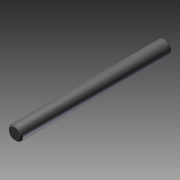
# Autodesk Inventor part: HHPMGS5pin
Saved by Autodesk Inventor 2011 SP1 (Build 150282100, 282)
## iProperties
Created: 2015-01-26
Part Number: HHPMGS5pin
Catalog Web Link: www.cadenas.de
Description: HHPMGS_pin-Low Dust Raise Hinges - Pin
Vendor: MISUMI
Document SubType Name: Modeling
Designer: PARTuser1
Manufacturer: MISUMI
Mass: 1.05662 g
Surface Area: 8.77648 cm^2
Volume: 1.05662 cm^3
Density: 1 g/cm^3
Category: PARTsolutions
Company: MISUMI
Title: HHPMGS5pin
Author: Cadenas PARTsolutions
Comments: Low Dust Raise Hinges - Pin
PSOL_IDENT_0: {\\10.0.0.236\data_v8\23d-libs\misumi\metric\39_accessories_for_al_extrusions\hhpmgs_pin.prj},166 {V
PSOL_IDENT_1: TYP=3D},{NB=HHPMGS5pin},{LINA=HHPMGS5pin},{NN=HHPMGS_pin},{DATE=17.11.2014 05:31:03},{GEOMDATE=10.08
PSOL_IDENT_2: .2009 08:47:00},{VERSION=},{LINEID=10},{LINESUBID=-1},{WBVAR=}  {NB=HHPMGS5pin},{LINA=HHPMGS5pin},{K
PSOL_IDENT_3: T=DUMMY},{PN=HHPMGS5},{TYPE=HHPMGS},{NO=5},{L=47}
SUPPLIER: MISUMI
ARTICLENO: HHPMGS5pin
BOMINFO: HHPMGS5pin
CREATOR: CADENAS GmbH
Autodesk Inventor part; units mm, degrees
ref_plane "YZ Plane" through (0, 0, 0) normal (1, 0, 0) x (0, 1, 0)
ref_plane "XZ Plane" through (0, 0, 0) normal (0, 1, 0) x (-1, 0, 0)
ref_plane "XY Plane" through (0, 0, 0) normal (0, 0, 1) x (1, 0, 0)
sketch "Sketch_1" plane through (0, 0, 0) normal (0, 0, 1) x (1, 0, 0)
  line L0 (0, -27) -> (0, 27)
  line L1 (0, 27) -> (2, 27)
  line L2 (2, 27) -> (2.5, 26.5)
  line L3 (2.5, 26.5) -> (2.5, -26.5)
  line L4 (2.5, -26.5) -> (2, -27)
  line L5 (2, -27) -> (0, -27)
  line L6 (0, -27) -> (0, 27)
  constraints: 14 end point
revolve "Revolution1" add sketch "Sketch_1" angle 360 about axis through (0, -27, 0) along (0, -1, 0)
ref_plane "cp_XY" through (0, 0, 0) normal (0, -1, 0) x (1, 0, 0)
ref_plane "cp_YZ" through (0, 0, 0) normal (1, 0, 0) x (0, 0, 1)
ref_plane "cp_ZX" through (0, 0, 0) normal (0, 0, 1) x (0, -1, 0)
body "Solid1"
